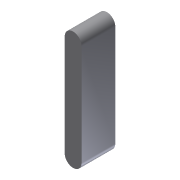
# Autodesk Inventor part: ShooterAcceleratorConcept
Saved by Autodesk Inventor 2012 (Build 160160000, 160)
## iProperties
Created: 2012-01-09
Part Number: ShooterAcceleratorConcept
Material: Default
Document SubType Name: Modeling
Designer: JesseK
Density: 1 g/cm^3
Author: JesseK
Autodesk Inventor part; units mm, degrees
ref_plane "YZ Plane" through (0, 0, 0) normal (1, 0, 0) x (0, 1, 0)
ref_plane "XZ Plane" through (0, 0, 0) normal (0, 1, 0) x (-1, 0, 0)
ref_plane "XY Plane" through (0, 0, 0) normal (0, 0, 1) x (1, 0, 0)
sketch "Sketch1" plane through (0, 0, 0) normal (0, 0, 1) x (1, 0, 0)
  arc A0 (-25.4, 0) -> (25.4, 0) centre (0, 0) ccw
  arc A1 (25.4, 304.8) -> (-25.4, 304.8) centre (0, 304.8) ccw
  line L0 (25.4, 304.8) -> (25.4, 0)
  line L1 (-25.4, 304.8) -> (-25.4, 0)
  dimension "d0" = 25.4
  dimension "d1" = 304.8
  constraints: 4 end point, 4 point on circle, 4 tangent, 2 centre point, 2 vertical, 1 coincident
  measures "d0" radius of A1
  measures "d1" distance of L0.start L0.end
extrude "Extrusion1" add sketch "Sketch1" along normal blind 101.6
body "Solid1"
